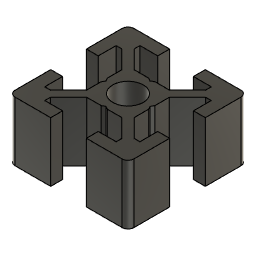
Doorbuffer (Autodesk Fusion 360 archive; units mm, degrees)
design "2020"
Autodesk Fusion 360 part; units mm, degrees
sketch "Sketch2" plane through (0, 0, 100) normal (0, 0, 1) x (-1, 0, 0)
  line L0 (8, 3) -> (10, 3)
  line L1 (10, 3) -> (10, 9)
  arc A0 (10, 9) -> (9, 10) centre (9, 9) ccw
  line L2 (9, 10) -> (3, 10)
  line L3 (3, 10) -> (3, 8)
  line L4 (3, 8) -> (6, 8)
  line L5 (6, 8) -> (6, 7.0607)
  line L6 (6, 7.0607) -> (2.9393, 4)
  line L7 (2.9393, 4) -> (0.5196, 4)
  line L8 (0.5196, 4) -> (0, 3.7)
  line L9 (0, 3.7) -> (-0.5196, 4)
  line L10 (-0.5196, 4) -> (-2.9393, 4)
  line L11 (-2.9393, 4) -> (-6, 7.0607)
  line L12 (-6, 7.0607) -> (-6, 8)
  line L13 (-6, 8) -> (-3, 8)
  line L14 (-3, 8) -> (-3, 10)
  line L15 (-3, 10) -> (-9, 10)
  arc A1 (-9, 10) -> (-10, 9) centre (-9, 9) ccw
  line L16 (-10, 9) -> (-10, 3)
  line L17 (-10, 3) -> (-8, 3)
  line L18 (-8, 3) -> (-8, 6)
  line L19 (-8, 6) -> (-7.0607, 6)
  line L20 (-7.0607, 6) -> (-4, 2.9393)
  line L21 (-4, 2.9393) -> (-4, 0.5196)
  line L22 (-4, 0.5196) -> (-3.7, 0)
  line L23 (-3.7, 0) -> (-4, -0.5196)
  line L24 (-4, -0.5196) -> (-4, -2.9393)
  line L25 (-4, -2.9393) -> (-7.0607, -6)
  line L26 (-7.0607, -6) -> (-8, -6)
  line L27 (-8, -6) -> (-8, -3)
  line L28 (-8, -3) -> (-10, -3)
  line L29 (-10, -3) -> (-10, -9)
  arc A2 (-10, -9) -> (-9, -10) centre (-9, -9) ccw
  line L30 (-9, -10) -> (-3, -10)
  line L31 (-3, -10) -> (-3, -8)
  line L32 (-3, -8) -> (-6, -8)
  line L33 (-6, -8) -> (-6, -7.0607)
  line L34 (-6, -7.0607) -> (-2.9393, -4)
  line L35 (-2.9393, -4) -> (-0.5196, -4)
  line L36 (-0.5196, -4) -> (0, -3.7)
  line L37 (0, -3.7) -> (0.5196, -4)
  line L38 (0.5196, -4) -> (2.9393, -4)
  line L39 (2.9393, -4) -> (6, -7.0607)
  line L40 (6, -7.0607) -> (6, -8)
  line L41 (6, -8) -> (3, -8)
  line L42 (3, -8) -> (3, -10)
  line L43 (3, -10) -> (9, -10)
  arc A3 (9, -10) -> (10, -9) centre (9, -9) ccw
  line L44 (10, -9) -> (10, -3)
  line L45 (10, -3) -> (8, -3)
  line L46 (8, -3) -> (8, -6)
  line L47 (8, -6) -> (7.0607, -6)
  line L48 (7.0607, -6) -> (4, -2.9393)
  line L49 (4, -2.9393) -> (4, -0.5196)
  line L50 (4, -0.5196) -> (3.7, 0)
  line L51 (3.7, 0) -> (4, 0.5196)
  line L52 (4, 0.5196) -> (4, 2.9393)
  line L53 (4, 2.9393) -> (7.0607, 6)
  line L54 (7.0607, 6) -> (8, 6)
  line L55 (8, 6) -> (8, 3)
  circle A4 centre (0, 0) radius 2.56
extrude "Extrude4" add sketch "Sketch2" along normal blind 470
extrude "Extrude5" cut 1 faces at (-7.6667, 8, 570) along direction (0, 0, -1) blind 460
move_body "Move1" bodies 1 to x (1, 0, 0) y (0, 1, 0) z (0, 0, 1) at (0, 0, -110)
equation "beam_length = 470 mm"
equation "d8 = beam_length"
equation "d6 = -beam_length + 30 mm"
